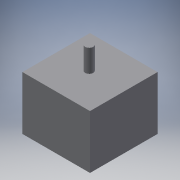
# Autodesk Inventor part: Motor
Saved by Autodesk Inventor 2016 (Build 200138000, 138)
## iProperties
Created: 2018-03-08
Part Number: Motor
Material: Generic
Document SubType Name: Modeling
Designer: Simon
Density: 1 g/cm^3
Appearance: Default
Author: Simon
Autodesk Inventor part; units mm, degrees
ref_plane "YZ Plane" through (0, 0, 0) normal (1, 0, 0) x (0, 1, 0)
ref_plane "XZ Plane" through (0, 0, 0) normal (0, 1, 0) x (-1, 0, 0)
ref_plane "XY Plane" through (0, 0, 0) normal (0, 0, 1) x (1, 0, 0)
sketch "Sketch1" plane through (0, 0, 0) normal (0, 0, 1) x (1, 0, 0)
  line L0 (0, 0) -> (42, 0)
  line L1 (42, 0) -> (42, 42)
  line L2 (42, 42) -> (0, 42)
  line L3 (0, 42) -> (0, 0)
  dimension "d0" = 42
  dimension "d1" = 42
  constraints: 8 end point, 2 parallel, 1 horizontal, 1 perpendicular
  measures "d0" distance of L2.end L1.end
  measures "d1" distance of L1.end L0.end
extrude "Extrusion1" add sketch "Sketch1" along normal blind 33.3
sketch "Sketch2" plane through (0, 0, 33.3) normal (0, 0, 1) x (1, 0, 0)
  circle A0 centre (21, 21) radius 2.5
  line L0 (42, 0) -> (42, 42) projected
  line L1 (42, 42) -> (0, 42) projected
  point P0 (0, 0)
  dimension "d4" = 5
  dimension "d7" = 21
  dimension "d8" = 21
  constraints: 1 centre point
  measures "d4" diameter of A0
  measures "d7" distance from line of L0 A0.centre
  measures "d8" distance from line of L1 A0.centre
extrude "Extrusion2" add sketch "Sketch2" along normal blind 16
body "Solid1"
